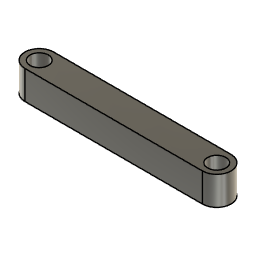
Fixed_Stick1_ver4 v1 (Autodesk Fusion 360 design; units mm, degrees)
Autodesk Fusion 360 part; units mm, degrees
sketch "스케치1" plane through (0, 0, 0) normal (0, 0, 1) x (1, 0, 0)
  line L0 (-25, -2.5) -> (6, -2.5)
  arc A0 (6, -2.5) -> (6, 2.5) centre (6, 0) ccw
  line L1 (6, 2.5) -> (-25, 2.5)
  arc A1 (-25, 2.5) -> (-25, -2.5) centre (-25, 0) ccw
  line L2 (-25, 0) -> (6, 0) construction
  circle A2 centre (6, 0) radius 1.6
  circle A3 centre (-25, 0) radius 1.6
  dimension "d1" = 31
  dimension "d2" = 5
  dimension "d3" = 3.2
  dimension "d4" = 3.2
  constraint tangent L0 A0
  constraint tangent A0 L1
  constraint parallel L0 L1
  constraint tangent L1 A1
  constraint tangent L0 A1
  constraint horizontal L2
  constraint concentric A0 A2
  constraint concentric A1 A3
  measures "d1" distance of A1.centre A0.centre
  measures "d2" diameter of A0
  measures "d3" diameter of A2
  measures "d4" diameter of A3
extrude "돌출1" add sketch "스케치1" along normal blind 5
